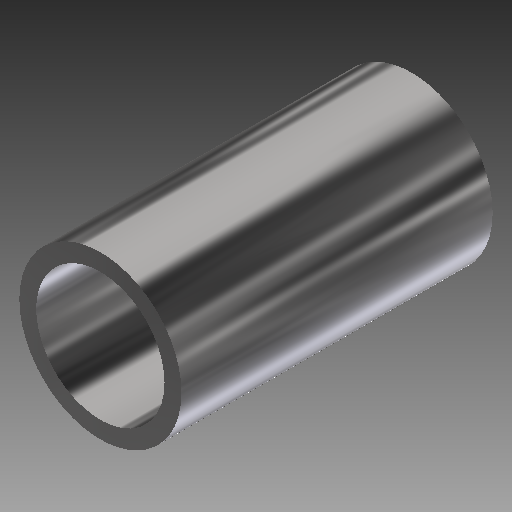
# Autodesk Inventor part: Separator
Saved by Autodesk Inventor 2017 (Build 210142000, 142)
## iProperties
Created: 2015-12-01
Part Number: Separator
Material: Stal, węglowa
Document SubType Name: Modeling
Designer: graaapsik
Density: 7.87 g/cm^3
Appearance: Częściowo polerowany
Mass: 22.6168 g
Surface Area: 33.6728 cm^2
Volume: 2.8738 cm^3
Author: graaapsik
Autodesk Inventor part; units mm, degrees
ref_plane "YZ Plane" through (0, 0, 0) normal (1, 0, 0) x (0, 1, 0)
ref_plane "XZ Plane" through (0, 0, 0) normal (0, 1, 0) x (-1, 0, 0)
ref_plane "XY Plane" through (0, 0, 0) normal (0, 0, 1) x (1, 0, 0)
sketch "Szkic1" plane through (0, 0, 0) normal (0, 0, 1) x (1, 0, 0)
  circle A0 centre (0, 0) radius 8.6
  dimension "d0" = 17.2
  constraints: 1 centre point, 1 coincident
  measures "d0" diameter of A0
extrude "Wyciągnięcie proste1" add sketch "Szkic1" along normal mid plane 33
sketch "Szkic2" plane through (0, 0, 16.5) normal (0, 0, 1) x (1, 0, 0)
  circle A0 centre (0, 0) radius 8.6 projected
hole "Otwór1" at (0, 0, 16.5) direction (0, 0, -1) diameter 13.6 end through all
